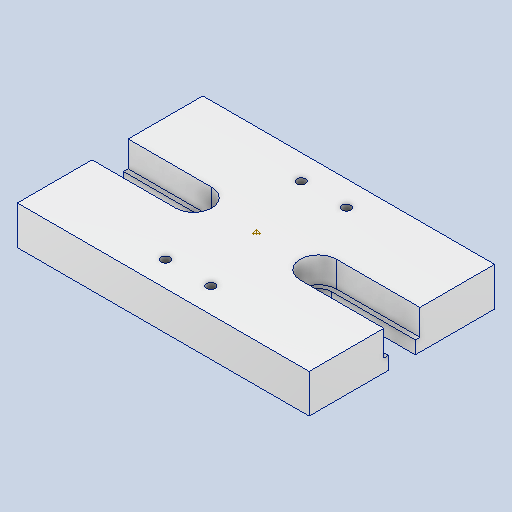
# Autodesk Inventor part: bottomblock_al_ledgereod
Saved by Autodesk Inventor 2024.2 (Build 282272000, 272)
## iProperties
Created: 2023-03-07
Part Number: bottomblock_al_ledgereod
Material: Aluminum 6061
Document SubType Name: Modeling
Designer: warke
Density: 2.7 g/cm^3
Appearance: Aluminum - Flat
Author: warke
Autodesk Inventor part; units mm, degrees
ref_plane "YZ Plane" through (0, 0, 0) normal (1, 0, 0) x (0, 1, 0)
ref_plane "XZ Plane" through (0, 0, 0) normal (0, 1, 0) x (-1, 0, 0)
ref_plane "XY Plane" through (0, 0, 0) normal (0, 0, 1) x (1, 0, 0)
sketch "Sketch1" plane through (0, 0, 0) normal (0, 1, 0) x (-1, 0, 0)
  line L0 (22.9489, 20.701) -> (-22.9489, 20.701)
  line L1 (-22.9489, 20.701) -> (-22.9489, -20.701)
  line L2 (-22.9489, -20.701) -> (22.9489, -20.701)
  line L3 (22.9489, -20.701) -> (22.9489, 20.701)
  line L4 (22.9489, 20.701) -> (-22.9489, -20.701) construction
  line L5 (-22.9489, 20.701) -> (22.9489, -20.701) construction
  point P0 (0, 0)
  dimension "d0" = 45.8978
  dimension "d1" = 41.402
  constraints: 12 end point, 2 midpoint, 2 parallel, 1 horizontal, 1 perpendicular
  measures "d0" distance of L2.end L1.end
  measures "d1" distance of L1.end L0.end
extrude "Extrusion1" add sketch "Sketch1" along normal blind 9.525
hole "Hole1" at (0, 0, 0) direction (0, 1, 0) diameter 4.9784 depth 6.35 thread size "1/4-20 UNC" class "2B" standard "ANSI Unified Screw Threads"
sketch "Sketch11" plane through (-22.9489, 0, 20.701) normal (0, 0, 1) x (1, 0, 0)
  line L0 (45.8978, 9.525) -> (0, 9.525) projected
  line L1 (45.8978, 0) -> (0, 0) projected
  line L2 (0, 9.525) -> (45.8978, 9.525)
  line L3 (45.8978, 9.525) -> (45.8978, 0)
  line L4 (45.8978, 0) -> (0, 0)
  line L5 (0, 0) -> (0, 9.525)
  point P0 (22.9489, 0)
  constraints: 8 end point, 2 parallel, 1 horizontal, 1 perpendicular
extrude "Extrusion6" cut sketch "Sketch11" against normal blind 3.175
sketch "Sketch12" plane through (22.9489, 0, -20.701) normal (0, 0, -1) x (-1, 0, 0)
  line L0 (0, 9.525) -> (45.8978, 9.525) projected
  line L1 (45.8978, 0) -> (45.8978, 9.525) projected
  line L2 (0, 9.525) -> (45.8978, 9.525)
  line L3 (45.8978, 9.525) -> (45.8978, 0)
  line L4 (45.8978, 0) -> (0, 0)
  line L5 (0, 0) -> (0, 9.525)
  point P0 (22.9489, 0)
  constraints: 8 end point, 2 parallel, 1 horizontal, 1 perpendicular
extrude "Extrusion7" cut sketch "Sketch12" against normal blind 3.175
sketch "Sketch13" plane through (22.9489, 0, 17.526) normal (1, 0, 0) x (0, 0, -1)
  line L0 (0, 9.525) -> (0, 0) projected
  line L1 (35.052, 0) -> (0, 0) projected
  line L2 (0, 9.525) -> (35.052, 9.525)
  line L3 (35.052, 9.525) -> (35.052, 0)
  line L4 (35.052, 0) -> (0, 0)
  line L5 (0, 0) -> (0, 9.525)
  point P0 (17.526, 0)
  constraints: 8 end point, 2 parallel, 1 horizontal, 1 perpendicular
extrude "Extrusion8" add sketch "Sketch13" along normal blind 12.9426
sketch "Sketch14" plane through (-22.9489, 0, 17.526) normal (-1, 0, 0) x (0, 0, 1)
  line L0 (-35.052, 9.525) -> (0, 9.525) projected
  line L1 (-35.052, 9.525) -> (0, 9.525)
  line L2 (0, 9.525) -> (0, 0)
  line L3 (0, 0) -> (-35.052, 0)
  line L4 (-35.052, 0) -> (-35.052, 9.525)
  point P0 (-17.526, 0)
  constraints: 8 end point, 2 parallel, 1 horizontal, 1 perpendicular
extrude "Extrusion9" add sketch "Sketch14" along normal blind 12.9426
sketch "Sketch2" plane through (0, 9.525, 0) normal (0, 1, 0) x (1, 0, 0)
  line L0 (22.9489, -20.701) -> (22.9489, 20.701) projected
  line L1 (-22.9489, -20.701) -> (22.9489, -20.701) projected
  line L2 (22.9489, 20.701) -> (-22.9489, 20.701) projected
  line L3 (-22.9489, 20.701) -> (-22.9489, -20.701) projected
  arc A0 (-15.3289, -3.302) -> (-15.3289, 3.302) centre (-15.3289, 0) ccw
  line L4 (-15.3289, -3.302) -> (-22.9489, -3.302)
  line L5 (-15.3289, 3.302) -> (-22.9489, 3.302)
  arc A1 (15.3289, 3.302) -> (15.3289, -3.302) centre (15.3289, 0) ccw
  line L6 (15.3289, 3.302) -> (22.9489, 3.302)
  line L7 (15.3289, -3.302) -> (22.9489, -3.302)
  line L8 (-22.9489, 4.445) -> (-15.3289, 4.445)
  arc A2 (-15.3289, -4.445) -> (-15.3289, 4.445) centre (-15.3289, 0) ccw
  line L9 (-15.3289, -4.445) -> (-22.9489, -4.445)
  line L10 (22.9489, 4.445) -> (15.3289, 4.445)
  arc A3 (15.3289, 4.445) -> (15.3289, -4.445) centre (15.3289, 0) ccw
  line L11 (15.3289, -4.445) -> (22.9489, -4.445)
  line L12 (22.9489, -4.445) -> (35.8915, -4.445)
  line L13 (35.8915, -17.526) -> (35.8915, 17.526) projected
  line L14 (22.9489, -3.302) -> (35.8915, -3.302)
  line L15 (22.9489, 3.302) -> (35.8915, 3.302)
  line L16 (22.9489, 4.445) -> (35.8915, 4.445)
  line L17 (-22.9489, 4.445) -> (-35.8915, 4.445)
  line L18 (-35.8915, -17.526) -> (-35.8915, 17.526) projected
  line L19 (-22.9489, 3.302) -> (-25.4, 3.302)
  line L20 (-22.9489, -3.302) -> (-35.8915, -3.302)
  line L21 (-22.9489, -4.445) -> (-35.8915, -4.445)
  line L22 (-25.4, 3.302) -> (-35.8915, 3.302)
  point P0 (22.9489, 0)
  point P1 (-22.9489, 0)
  dimension "d21" = 1.143
  constraints: 34 end point, 12 point on line, 8 point on circle, 6 perpendicular, 4 centre point, 4 parallel, 3 horizontal, 3 tangent, 2 midpoint, 4 other
  measures "d21" distance between parallel lines of L6 L10
extrude "Extrusion10" cut sketch "Sketch2" against normal through all contours L7 A1 L6 L0 | L0 L15 L13 L14 | L20 L18 L22 L19 L3 | L3 L5 A0 L4
extrude "Extrusion11" cut sketch "Sketch2" against normal blind 6.35 contours L11 A3 L10 L0 L6 A1 L7 | L0 L14 L13 L12 | L21 L18 L20 L3 | L3 L4 A0 L5 L8 A2 L9 | L0 L16 L13 L15 | L19 L22 L18 L17 L3
sketch "Sketch15" plane through (22.9489, 0, -17.526) normal (0, 0, -1) x (-1, 0, 0)
  line L0 (-12.9426, 9.525) -> (-12.9426, 0) projected
  line L1 (58.8404, 9.525) -> (58.8404, 0) projected
  line L2 (-12.9426, 9.525) -> (58.8404, 9.525)
  line L3 (58.8404, 9.525) -> (58.8404, 0)
  line L4 (58.8404, 0) -> (-12.9426, 0)
  line L5 (-12.9426, 0) -> (-12.9426, 9.525)
  point P0 (22.9489, 0)
  constraints: 8 end point, 2 parallel, 1 horizontal, 1 perpendicular
extrude "Extrusion12" add sketch "Sketch15" along normal blind 5.285
sketch "Sketch16" plane through (-22.9489, 0, 17.526) normal (0, 0, 1) x (1, 0, 0)
  line L0 (-12.9426, 3.175) -> (-12.9426, 9.525) projected
  line L1 (58.8404, 0) -> (-12.9426, 0) projected
  line L2 (-12.9426, 9.525) -> (58.8404, 9.525)
  line L3 (58.8404, 9.525) -> (58.8404, 0)
  line L4 (58.8404, 0) -> (-12.9426, 0)
  line L5 (-12.9426, 0) -> (-12.9426, 9.525)
  point P0 (22.9489, 0)
  constraints: 8 end point, 2 parallel, 1 horizontal, 1 perpendicular
extrude "Extrusion13" add sketch "Sketch16" along normal blind 5.285
sketch "Sketch19" plane through (0, 9.525, 0) normal (0, 1, 0) x (1, 0, 0)
  line L0 (-35.8915, 3.302) -> (-35.8915, 22.811) projected
  line L1 (-35.8915, 22.811) -> (-5.5893, 22.811)
  line L2 (-35.8915, 16.6642) -> (-35.8915, 22.811)
  line L3 (35.8915, 22.811) -> (-35.8915, 22.811) projected
  line L4 (35.8915, 22.811) -> (5.5893, 22.811)
  line L5 (35.8915, 16.6642) -> (35.8915, 22.811)
  line L6 (35.8915, -22.811) -> (-35.8915, -22.811) projected
  line L7 (-35.8915, -22.811) -> (-5.5893, -22.811)
  line L8 (-35.8915, -16.6642) -> (-35.8915, -22.811)
  line L9 (35.8915, -22.811) -> (5.5893, -22.811)
  line L10 (35.8915, -16.6642) -> (35.8915, -22.811)
  point P0 (0, 0)
  point P1 (-5.5893, 16.6642)
  point P2 (5.5893, 16.6642)
  point P3 (-5.5893, -16.6642)
  point P4 (5.5893, -16.6642)
  constraints: 16 end point, 4 horizontal, 1 point on line
hole "Hole2" at (-5.5893, 9.525, 16.6642) at (5.5893, 9.525, 16.6642) at (-5.5893, 9.525, -16.6642) at (5.5893, 9.525, -16.6642) direction (0, -1, 0) diameter 2.1565 depth 6.35 thread size "4-40 UNC" class "2B" standard "ANSI Unified Screw Threads"
body "Solid1"
